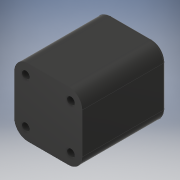
# Autodesk Inventor part: 2point_linear_connector
Saved by Autodesk Inventor 2019.4 (Build 234330000, 330)
## iProperties
Created: 2020-10-12
Part Number: 2point_linear_connector
Material: Generic
Document SubType Name: Modeling
Designer: deanv
Density: 1 g/cm^3
Appearance: Smooth - Black
Author: deanv
Autodesk Inventor part; units mm, degrees
ref_plane "YZ Plane" through (0, 0, 0) normal (1, 0, 0) x (0, 1, 0)
ref_plane "XZ Plane" through (0, 0, 0) normal (0, 1, 0) x (-1, 0, 0)
ref_plane "XY Plane" through (0, 0, 0) normal (0, 0, 1) x (1, 0, 0)
sketch "Sketch1" plane through (0, 0, 0) normal (0, 0, 1) x (1, 0, 0)
  line L0 (-10, -10) -> (10, -10) construction
  line L1 (10, -10) -> (10, 10) construction
  line L2 (10, 10) -> (-10, 10) construction
  line L3 (-10, 10) -> (-10, -10) construction
  line L4 (-10, -10) -> (10, 10) construction
  line L5 (10, -10) -> (-10, 10) construction
  line L6 (15, -15) -> (-15, -15)
  line L7 (-15, -15) -> (-15, 15)
  line L8 (-15, 15) -> (15, 15)
  line L9 (15, 15) -> (15, -15)
  line L10 (15, -15) -> (-15, 15) construction
  line L11 (-15, -15) -> (15, 15) construction
  line L12 (10, -10) -> (-10, -10)
  line L13 (-10, -10) -> (-10, 10)
  line L14 (-10, 10) -> (10, 10)
  line L15 (10, 10) -> (10, -10)
  line L16 (10, -10) -> (-10, 10) construction
  line L17 (-10, -10) -> (10, 10) construction
  point P0 (0, 0)
  dimension "d0" = 20
  dimension "d1" = 20
  dimension "d2" = 30
  dimension "d3" = 30
  constraints: 36 end point, 6 midpoint, 6 parallel, 4 coincident, 3 horizontal, 3 perpendicular
  measures "d0" distance of L2.end L1.end
  measures "d1" distance of L1.end L0.end
  measures "d2" distance of L7.end L8.end
  measures "d3" distance of L6.end L7.end
extrude "Extrusion1" add sketch "Sketch1" along normal blind 37 contours L6 L7 L8 L9 | L12 L13 L14 L15
extrude "Extrusion2" cut sketch "Sketch1" along normal blind 26 contours L12 L13 L14 L15
hole "Hole1" at (-10, 10, 0) at (10, 10, 0) at (10, -10, 0) at (-10, -10, 0) direction (0, 0, 1) diameter 3.5 end through all counterbore diameter 6 counterbore depth 30
fillet "Fillet1" radius 6 4 edges at (15, -15, 18.5) (15, 15, 18.5) (-15, 15, 18.5) (-15, -15, 18.5)
fillet "Fillet2" radius 1 8 edges at (7, 10, 13) (-7, 10, 13) (10, -7, 13) (-10, -7, 13) (10, 7, 13) (-10, 7, 13) (7, -10, 13) (-7, -10, 13)
fillet "Fillet3" radius 1 8 edges at (-13.2426, 13.2426, 0) (0, 15, 0) (13.2426, 13.2426, 0) (15, 0, 0) (13.2426, -13.2426, 0) (0, -15, 0) (-13.2426, -13.2426, 0) (-15, 0, 0)
equation "\"d3\" = d2"
body "Solid1"
